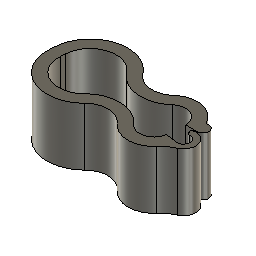
can_cable_ptfe_clip (Autodesk Fusion 360 design; units mm, degrees)
Autodesk Fusion 360 part; units mm, degrees
sketch "Sketch1" plane through (0, 0, 0) normal (0, 0, 1) x (1, 0, 0)
  line L0 (1.75, 0) -> (22.5, 0)
  arc A0 (2.5867, 1.9676) -> (5.5063, 1.6827) centre (4.1786, 3.1784) ccw
  arc A1 (2.5867, 1.9676) -> (-3.25, 0) centre (0, 0) ccw
  arc A2 (9.25, 0) -> (5.5063, 1.6827) centre (7, 0) ccw
  line L1 (0, 0) -> (-9.754, 0) construction
  line L2 (-0.0298, -0.4392) -> (6.906, -1.3851) construction
  line L3 (-0.0298, -0.4392) -> (-3.25, 0) construction
  arc A3 (-3.25, 0) -> (2.2673, -2.7382) centre (-0.0298, -0.4392) ccw
  arc A4 (5.1986, -2.8504) -> (2.2673, -2.7382) centre (3.681, -4.153) ccw
  arc A5 (5.1986, -2.8504) -> (9.1354, -1.6891) centre (6.906, -1.3851) ccw
  line L4 (6.906, -1.3851) -> (14.4668, -2.4162) construction
  line L5 (9.25, 0) -> (9.25, 1.1887) construction
  line L6 (9.1354, -1.6891) -> (9.284, -0.5992) construction
  line L7 (9.284, -0.5992) -> (9.3516, -0.1038)
  arc A6 (9.0126, -2.1755) -> (9.3516, -0.1038) centre (9.2097, -1.1441) ccw
  arc A7 (9.1354, -1.6891) -> (9.284, -0.5992) centre (9.2097, -1.1441) ccw
  arc A8 (9.25, 0) -> (9.0382, 0.9529) centre (9.25, 0.5) ccw
  line L8 (9.1354, -1.6891) -> (8.1445, -1.554)
  circle A9 centre (6.906, -1.3851) radius 2.25
  circle A10 centre (9.2097, -1.1441) radius 0.55
  circle A11 centre (9.2097, -1.1441) radius 1.05
  arc A12 (8.2852, -0.6486) -> (8.3822, -1.0313) centre (9.284, -0.5992) ccw
  arc A13 (8.3822, -1.0313) -> (8.1445, -1.554) centre (9.1354, -1.6891) ccw
  arc A14 (5.9575, -2.1992) -> (8.1445, -1.554) centre (6.906, -1.3851) ccw
  arc A15 (5.9575, -2.1992) -> (1.5605, -2.0308) centre (3.681, -4.153) ccw
  arc A16 (-2.249, -0.0679) -> (1.5605, -2.0308) centre (-0.0298, -0.4392) ccw
  arc A17 (1.7908, 1.3622) -> (-2.249, -0.0679) centre (0, 0) ccw
  arc A18 (1.7908, 1.3622) -> (6.1702, 0.9348) centre (4.1786, 3.1784) ccw
  arc A19 (8.1411, -0.5102) -> (6.1702, 0.9348) centre (7, 0) ccw
  arc A20 (8.1411, -0.5102) -> (8.2852, -0.6486) centre (9.25, 0.5) ccw
  arc A21 (8.8249, -3.1577) -> (10.7264, 0.235) centre (9.2097, -1.1441) ccw
  arc A22 (10.7264, 0.235) -> (8.6147, 1.8588) centre (9.25, 0.5) ccw
  dimension "d1" = 6.5
  dimension "d2" = 4.5
  dimension "d3" = 4
  dimension "d4" = 7
  dimension "d9" = 7
  dimension "d10" = 1
  dimension "d11" = 1.1
  dimension "d12" = 0.5
  dimension "d13" = -1
  constraint coincident A1.centre L1.start
  constraint coincident A2.centre L0
  constraint tangent A0 A1
  constraint tangent A0 A2
  constraint horizontal L1
  constraint coincident L1 A1.end
  constraint coincident L0 A2.start
  constraint equal A1 A3
  constraint equal A0 A4
  constraint equal A2 A5
  constraint tangent A3 A4
  constraint tangent A4 A5
  constraint coincident L2.start L3.start
  constraint coincident L2.end A5.centre
  constraint collinear L2 L3
  constraint parallel L2 L4
  constraint tangent A2 L5
  constraint coincident A8.centre L5
  constraint coincident L4 A5.end
  constraint tangent A5 L6
  constraint midpoint L6 A6.centre
  constraint tangent L4 A7
  constraint perpendicular L4 L7
  constraint concentric A6 A7
  constraint coincident A5 A6.start
  constraint coincident A2 A8.end
  constraint tangent A7 L8
  constraint concentric A5 A9
  constraint concentric A7 A10
  constraint concentric A6 A11
  measures "d1" diameter of A1
  measures "d2" diameter of A2
  measures "d3" diameter of A0
  measures "d4" distance of A1.centre A2.centre
  measures "d9" distance of L2.start L2.end
  measures "d10" diameter of A8
  measures "d11" diameter of A7
  measures "d12" distance of L6.end L7.end
extrude "Extrude1" add sketch "Sketch1" along normal blind 5 contours L0 A9 A19 | L0 A0 A1 A2 A3 A4 A9 A15 A16 A17 A18 A19 | A5 L8 A9 A11 A14 A15 | A2 A8 | L7 A9 A10 A11 | A5 L8 A9 A11 | A5 L7 A6 A7 A9 A10 A11 picked at (8.4833, 0.0606)
scale "Scale1" factor 1.6 about (-3.25, 0, 5) bodies 1
fillet "Fillet1" radius 278 1 edges at (-3.25, 0, 1)
fillet "Fillet1" radius 506.5 1 edges at (-1.6484, -0.1087, 1)
fillet "Fillet1" radius 4.5 1 edges at (16.3701, -3.4808, 1)
fillet "Fillet1" radius 0.3 1 edges at (16.4112, 1.5247, 1)
fillet "Fillet1" radius 0.3 2 edges at (16.0356, -0.2814, 1) (16.3887, -1.0022, 1)
equation "d9 = d4"
equation "d11 = d10 + 0.1 mm"
